Autodesk Inventor part; units mm, degrees
(part 6 of 10)
  spline S17 degree 5 poles (-10.8792, 7.6525) (-10.8768, 7.6467) (-10.8736, 7.6389) (-10.8696, 7.6293) (-10.8648, 7.6178) (-10.8591, 7.6044) (-10.855, 7.5949) (-10.8509, 7.5854) (-10.8468, 7.576) (-10.8427, 7.5666) (-10.8386, 7.5572) (-10.8344, 7.5479) (-10.8303, 7.5386) (-10.8261, 7.5293) (-10.8219, 7.5201) (-10.8177, 7.5109) (-10.8135, 7.5017) (-10.8093, 7.4926) (-10.8051, 7.4835) (-10.8008, 7.4745) (-10.7966, 7.4654) (-10.7923, 7.4565) (-10.788, 7.4475) (-10.7838, 7.4386) (-10.7795, 7.4297) (-10.7751, 7.4209) (-10.7708, 7.4121) (-10.7665, 7.4033) (-10.7621, 7.3946) (-10.7578, 7.3859) (-10.7526, 7.3755) (-10.7473, 7.3651) (-10.742, 7.3548) (-10.7359, 7.3429) (-10.7297, 7.331) (-10.7244, 7.3209) (-10.7191, 7.3109) (-10.7137, 7.3009) (-10.7084, 7.2909) (-10.703, 7.281) (-10.6977, 7.2712) (-10.6914, 7.2597) (-10.6851, 7.2484) (-10.6797, 7.2387) (-10.6734, 7.2275) (-10.667, 7.2164) (-10.6616, 7.2069) (-10.6552, 7.1959) (-10.6489, 7.185) (-10.6434, 7.1757) (-10.6361, 7.1633) (-10.6288, 7.1511) (-10.6224, 7.1405) (-10.6159, 7.13) (-10.6077, 7.1165) (-10.6012, 7.1061) (-10.5948, 7.0959) (-10.5883, 7.0856) (-10.58, 7.0726) (-10.5736, 7.0626) (-10.5671, 7.0526) (-10.5597, 7.0413) (-10.5523, 7.0301) (-10.5467, 7.0218) (-10.5402, 7.0121) (-10.5338, 7.0026) (-10.5282, 6.9944) (-10.5217, 6.985) (-10.5152, 6.9757) (-10.5097, 6.9677) (-10.5032, 6.9585) (-10.4967, 6.9494) (-10.4911, 6.9416) (-10.4846, 6.9326) (-10.4782, 6.9237) (-10.4726, 6.9162) (-10.4662, 6.9074) (-10.4597, 6.8987) (-10.4542, 6.8914) (-10.4477, 6.8828) (-10.4413, 6.8744) (-10.4357, 6.8672) (-10.4293, 6.8589) (-10.4229, 6.8507) (-10.4174, 6.8437) (-10.411, 6.8356) (-10.4046, 6.8277) (-10.3991, 6.8209) (-10.3928, 6.813) (-10.3864, 6.8053) (-10.381, 6.7987) (-10.3747, 6.7911) (-10.3684, 6.7835) (-10.363, 6.7772) (-10.3567, 6.7698) (-10.3504, 6.7625) (-10.3451, 6.7563) (-10.3389, 6.7491) (-10.3326, 6.7421) (-10.3273, 6.7361) (-10.3212, 6.7292) (-10.315, 6.7223) (-10.3098, 6.7166) (-10.3037, 6.7099) (-10.2976, 6.7033) (-10.2924, 6.6977) (-10.2864, 6.6912) (-10.2804, 6.6849) (-10.2753, 6.6795) (-10.2693, 6.6733) (-10.2634, 6.6672) (-10.2583, 6.662) (-10.2525, 6.656) (-10.2467, 6.6501) (-10.2417, 6.6451) (-10.2359, 6.6394) (-10.2302, 6.6338) (-10.2253, 6.629) (-10.2196, 6.6235) (-10.214, 6.6181) (-10.2092, 6.6135) (-10.2036, 6.6082) (-10.1981, 6.6031) (-10.1934, 6.5987) (-10.188, 6.5937) (-10.1826, 6.5887) (-10.178, 6.5846) (-10.1727, 6.5798) (-10.1674, 6.5751) (-10.163, 6.5711) (-10.1578, 6.5666) (-10.1527, 6.5621) (-10.1483, 6.5583) (-10.1433, 6.554) (-10.1383, 6.5498) (-10.1341, 6.5463) (-10.1292, 6.5422) (-10.1243, 6.5382) (-10.1203, 6.5349) (-10.1155, 6.531) (-10.1109, 6.5273) (-10.1069, 6.5241) (-10.1024, 6.5205) (-10.0979, 6.517) (-10.0941, 6.5141) (-10.0898, 6.5107) (-10.0855, 6.5075) (-10.0818, 6.5047) (-10.0777, 6.5016) (-10.0736, 6.4986) (-10.0701, 6.496) (-10.0662, 6.4931) (-10.0623, 6.4903) (-10.059, 6.488) (-10.0558, 6.4857) (-10.0516, 6.4828) (-10.048, 6.4803) (-10.044, 6.4775) (-10.0401, 6.4749) (-10.0363, 6.4724) (-10.0336, 6.4706) (-10.0309, 6.4688) (-10.0287, 6.4674) (-10.0266, 6.466) (-10.0245, 6.4646) (-10.0224, 6.4633) (-10.0204, 6.4621) (-10.0185, 6.4608) (-10.0166, 6.4597) (-10.0147, 6.4585) (-10.0129, 6.4574) (-10.0112, 6.4564) (-10.0095, 6.4553) (-10.0078, 6.4544) (-10.0063, 6.4534) (-10.0047, 6.4525) (-10.0033, 6.4517) (-10.0018, 6.4508) (-10.0005, 6.4501) (-9.9992, 6.4493) (-9.9979, 6.4486) (-9.9967, 6.448) (-9.9956, 6.4473) (-9.9946, 6.4468) (-9.9936, 6.4462) (-9.9926, 6.4457) (-9.9918, 6.4452) (-9.9909, 6.4448) (-9.9902, 6.4444) (-9.9895, 6.4441) (-9.9889, 6.4438) (-9.9883, 6.4434) (-9.9878, 6.4432) (-9.9875, 6.443) (-9.9873, 6.4429) (-9.9872, 6.4429) knots -1 -1 -1 -1 -1 -1 -0.9875 -0.983333 -0.979167 -0.975 -0.970833 -0.966667 -0.9625 -0.958333 -0.954167 -0.95 -0.945833 -0.941667 -0.9375 -0.933333 -0.929167 -0.925 -0.920833 -0.916667 -0.9125 -0.908333 -0.904167 -0.9 -0.895833 -0.891667 -0.8875 -0.883333 -0.879167 -0.875 -0.870833 -0.8625 -0.858333 -0.854167 -0.845833 -0.841667 -0.8375 -0.833333 -0.829167 -0.820833 -0.816667 -0.8125 -0.804167 -0.8 -0.795833 -0.7875 -0.783333 -0.779167 -0.770833 -0.766667 -0.7625 -0.75 -0.745833 -0.741667 -0.7375 -0.725 -0.720833 -0.716667 -0.7125 -0.7 -0.695833 -0.691667 -0.683333 -0.679167 -0.675 -0.666667 -0.6625 -0.658333 -0.65 -0.645833 -0.641667 -0.633333 -0.629167 -0.625 -0.616667 -0.6125 -0.608333 -0.6 -0.595833 -0.591667 -0.583333 -0.579167 -0.575 -0.566667 -0.5625 -0.558333 -0.55 -0.545833 -0.541667 -0.533333 -0.529167 -0.525 -0.516667 -0.5125 -0.508333 -0.5 -0.495833 -0.491667 -0.483333 -0.479167 -0.475 -0.466667 -0.4625 -0.458333 -0.45 -0.445833 -0.441667 -0.433333 -0.429167 -0.425 -0.416667 -0.4125 -0.408333 -0.4 -0.395833 -0.391667 -0.383333 -0.379167 -0.375 -0.366667 -0.3625 -0.358333 -0.35 -0.345833 -0.341667 -0.333333 -0.329167 -0.325 -0.316667 -0.3125 -0.308333 -0.3 -0.295833 -0.291667 -0.283333 -0.279167 -0.275 -0.266667 -0.2625 -0.258333 -0.25 -0.245833 -0.241667 -0.233333 -0.229167 -0.225 -0.216667 -0.2125 -0.208333 -0.2 -0.195833 -0.191667 -0.183333 -0.179167 -0.175 -0.170833 -0.158333 -0.154167 -0.145833 -0.141667 -0.1375 -0.133333 -0.129167 -0.125 -0.120833 -0.116667 -0.1125 -0.108333 -0.104167 -0.1 -0.095833 -0.091667 -0.0875 -0.083333 -0.079167 -0.075 -0.070833 -0.066667 -0.0625 -0.058333 -0.054167 -0.05 -0.045833 -0.041667 -0.0375 -0.033333 -0.029167 -0.025 -0.020833 -0.016667 -0.0125 -0.008333 0 0 0 0 0 0
  line L36 (-8.4168, 7.2079) -> (-9.0752, 7.804)
  arc A18 (-7.5895, 7.9321) -> (-8.4168, 7.2079) centre (-4.8955, 4.02) ccw
  line L37 (-9.0752, 7.804) -> (-9.0757, 7.8044)
  spline S18 degree 5 poles (-9.0757, 7.8044) (-9.0757, 7.8045) (-9.0758, 7.8046) (-9.076, 7.8047) (-9.0763, 7.8049) (-9.0767, 7.8053) (-9.0771, 7.8057) (-9.0777, 7.8061) (-9.0782, 7.8066) (-9.0789, 7.8071) (-9.0796, 7.8077) (-9.0804, 7.8084) (-9.0812, 7.809) (-9.0821, 7.8097) (-9.083, 7.8105) (-9.084, 7.8113) (-9.0851, 7.8122) (-9.0862, 7.813) (-9.0874, 7.814) (-9.0886, 7.8149) (-9.0899, 7.8159) (-9.0913, 7.817) (-9.0927, 7.818) (-9.0942, 7.8191) (-9.0957, 7.8203) (-9.0973, 7.8215) (-9.0989, 7.8227) (-9.1006, 7.8239) (-9.1024, 7.8252) (-9.1042, 7.8265) (-9.1061, 7.8278) (-9.108, 7.8292) (-9.1104, 7.8309) (-9.1129, 7.8326) (-9.1154, 7.8343) (-9.1185, 7.8365) (-9.1217, 7.8386) (-9.1245, 7.8405) (-9.1279, 7.8427) (-9.1314, 7.845) (-9.1345, 7.8471) (-9.1376, 7.8491) (-9.1414, 7.8515) (-9.1464, 7.8547) (-9.1516, 7.8579) (-9.157, 7.8612) (-9.1625, 7.8646) (-9.1683, 7.868) (-9.1728, 7.8707) (-9.1775, 7.8734) (-9.1822, 7.8761) (-9.1878, 7.8793) (-9.1928, 7.8821) (-9.1972, 7.8846) (-9.2023, 7.8874) (-9.2076, 7.8903) (-9.2122, 7.8928) (-9.2176, 7.8957) (-9.2232, 7.8987) (-9.228, 7.9012) (-9.2338, 7.9042) (-9.2396, 7.9072) (-9.2447, 7.9098) (-9.2507, 7.9128) (-9.2568, 7.9159) (-9.2621, 7.9185) (-9.2684, 7.9216) (-9.2748, 7.9246) (-9.2803, 7.9273) (-9.2869, 7.9304) (-9.2935, 7.9335) (-9.2993, 7.9362) (-9.3061, 7.9393) (-9.313, 7.9424) (-9.319, 7.9451) (-9.3261, 7.9483) (-9.3333, 7.9514) (-9.3395, 7.9541) (-9.3468, 7.9572) (-9.3543, 7.9604) (-9.3607, 7.9631) (-9.3683, 7.9662) (-9.376, 7.9694) (-9.3827, 7.9721) (-9.3905, 7.9752) (-9.3985, 7.9784) (-9.4054, 7.981) (-9.4135, 7.9842) (-9.4217, 7.9873) (-9.4287, 7.99) (-9.4371, 7.9931) (-9.4455, 7.9962) (-9.4528, 7.9988) (-9.4614, 8.0019) (-9.4701, 8.005) (-9.4776, 8.0076) (-9.4865, 8.0107) (-9.4954, 8.0137) (-9.5031, 8.0163) (-9.5122, 8.0193) (-9.5213, 8.0223) (-9.5292, 8.0249) (-9.5385, 8.0279) (-9.5479, 8.0308) (-9.556, 8.0334) (-9.5656, 8.0363) (-9.5752, 8.0392) (-9.5835, 8.0417) (-9.5933, 8.0446) (-9.6031, 8.0474) (-9.6116, 8.0498) (-9.6216, 8.0527) (-9.6317, 8.0555) (-9.6404, 8.0578) (-9.6506, 8.0606) (-9.6609, 8.0633) (-9.6697, 8.0656) (-9.6802, 8.0683) (-9.6907, 8.071) (-9.6997, 8.0733) (-9.7104, 8.0759) (-9.7211, 8.0785) (-9.7303, 8.0807) (-9.7412, 8.0832) (-9.7521, 8.0857) (-9.7616, 8.0878) (-9.7726, 8.0903) (-9.7838, 8.0927) (-9.7934, 8.0948) (-9.8046, 8.0972) (-9.816, 8.0995) (-9.8257, 8.1015) (-9.8372, 8.1038) (-9.8488, 8.106) (-9.8587, 8.1079) (-9.8704, 8.1101) (-9.8821, 8.1123) (-9.8922, 8.1141) (-9.9041, 8.1162) (-9.916, 8.1182) (-9.9263, 8.12) (-9.9384, 8.122) (-9.9505, 8.1239) (-9.9609, 8.1256) (-9.9732, 8.1275) (-9.9855, 8.1293) (-9.9961, 8.1309) (-10.0103, 8.1329) (-10.0246, 8.1349) (-10.0372, 8.1366) (-10.0499, 8.1382) (-10.0626, 8.1398) (-10.0772, 8.1417) (-10.0918, 8.1434) (-10.1066, 8.1451) (-10.1215, 8.1467) (-10.1383, 8.1485) (-10.1495, 8.1496) (-10.1608, 8.1507) (-10.1759, 8.1522) (-10.1912, 8.1535) (-10.2045, 8.1547) (-10.218, 8.1558) (-10.2315, 8.1569) (-10.2411, 8.1576) (-10.2508, 8.1583) (-10.2606, 8.159) (-10.2703, 8.1596) (-10.2801, 8.1603) (-10.2899, 8.1609) (-10.2998, 8.1615) (-10.3097, 8.1621) (-10.3196, 8.1626) (-10.3295, 8.1631) (-10.3395, 8.1636) (-10.3494, 8.1641) (-10.3595, 8.1645) (-10.3695, 8.165) (-10.3796, 8.1654) (-10.3897, 8.1657) (-10.3998, 8.1661) (-10.41, 8.1664) (-10.4201, 8.1667) (-10.4304, 8.167) (-10.4406, 8.1672) (-10.4509, 8.1674) (-10.4611, 8.1676) (-10.4715, 8.1678) (-10.4818, 8.1679) (-10.4963, 8.1681) (-10.5088, 8.1682) (-10.5193, 8.1682) (-10.5276, 8.1683) (-10.5339, 8.1683) knots 0 0 0 0 0 0 0.004167 0.008333 0.0125 0.016667 0.020833 0.025 0.029167 0.033333 0.0375 0.041667 0.045833 0.05 0.054167 0.058333 0.0625 0.066667 0.070833 0.075 0.079167 0.083333 0.0875 0.091667 0.095833 0.1 0.104167 0.108333 0.1125 0.116667 0.120833 0.125 0.129167 0.1375 0.141667 0.145833 0.154167 0.158333 0.1625 0.170833 0.175 0.179167 0.183333 0.191667 0.208333 0.2125 0.216667 0.220833 0.229167 0.2375 0.241667 0.245833 0.254167 0.258333 0.2625 0.270833 0.275 0.279167 0.2875 0.291667 0.295833 0.304167 0.308333 0.3125 0.320833 0.325 0.329167 0.3375 0.341667 0.345833 0.354167 0.358333 0.3625 0.370833 0.375 0.379167 0.3875 0.391667 0.395833 0.404167 0.408333 0.4125 0.420833 0.425 0.429167 0.4375 0.441667 0.445833 0.454167 0.458333 0.4625 0.470833 0.475 0.479167 0.4875 0.491667 0.495833 0.504167 0.508333 0.5125 0.520833 0.525 0.529167 0.5375 0.541667 0.545833 0.554167 0.558333 0.5625 0.570833 0.575 0.579167 0.5875 0.591667 0.595833 0.604167 0.608333 0.6125 0.620833 0.625 0.629167 0.6375 0.641667 0.645833 0.654167 0.658333 0.6625 0.670833 0.675 0.679167 0.6875 0.691667 0.695833 0.704167 0.708333 0.7125 0.720833 0.725 0.729167 0.7375 0.741667 0.745833 0.754167 0.758333 0.7625 0.770833 0.775 0.779167 0.791667 0.795833 0.8 0.804167 0.808333 0.825 0.829167 0.833333 0.8375 0.845833 0.85 0.854167 0.866667 0.870833 0.875 0.879167 0.883333 0.8875 0.891667 0.895833 0.9 0.904167 0.908333 0.9125 0.916667 0.920833 0.925 0.929167 0.933333 0.9375 0.941667 0.945833 0.95 0.954167 0.958333 0.9625 0.966667 0.970833 0.975 0.979167 0.983333 0.9875 1 1 1 1 1 1
  arc A19 (-10.5339, 8.1683) -> (-10.8792, 7.6525) centre (-4.8955, 4.02) ccw
  arc A20 (-11.3072, 1.2111) -> (-11.0332, 0.6542) centre (-4.8955, 4.02) ccw
  line L38 (-9.417, 2.5644) -> (-10.2624, 2.2923)
  line L39 (-10.2624, 2.2923) -> (-10.263, 2.2921)
  spline S19 degree 5 poles (-10.263, 2.2921) (-10.2631, 2.292) (-10.2632, 2.292) (-10.2634, 2.2919) (-10.2638, 2.2918) (-10.2643, 2.2916) (-10.2648, 2.2914) (-10.2655, 2.2912) (-10.2662, 2.2909) (-10.267, 2.2906) (-10.2678, 2.2903) (-10.2688, 2.29) (-10.2698, 2.2896) (-10.2708, 2.2892) (-10.2719, 2.2888) (-10.2731, 2.2883) (-10.2744, 2.2878) (-10.2757, 2.2873) (-10.2771, 2.2867) (-10.2786, 2.2861) (-10.2801, 2.2855) (-10.2817, 2.2848) (-10.2833, 2.2841) (-10.285, 2.2834) (-10.2867, 2.2827) (-10.2886, 2.2819) (-10.2904, 2.281) (-10.2924, 2.2802) (-10.2943, 2.2793) (-10.2964, 2.2784) (-10.2985, 2.2774) (-10.3006, 2.2764) (-10.3033, 2.2752) (-10.306, 2.2739) (-10.3088, 2.2726) (-10.3122, 2.271) (-10.3156, 2.2693) (-10.3187, 2.2678) (-10.3223, 2.266) (-10.326, 2.2641) (-10.3293, 2.2625) (-10.3332, 2.2605) (-10.3372, 2.2584) (-10.3407, 2.2565) (-10.3449, 2.2543) (-10.3491, 2.252) (-10.3528, 2.25) (-10.3572, 2.2476) (-10.3617, 2.2451) (-10.3656, 2.2429) (-10.3703, 2.2403) (-10.375, 2.2376) (-10.3791, 2.2352) (-10.3839, 2.2324) (-10.3889, 2.2295) (-10.3932, 2.2269) (-10.3982, 2.2239) (-10.4034, 2.2208) (-10.4078, 2.218) (-10.4131, 2.2148) (-10.4184, 2.2114) (-10.423, 2.2085) (-10.4285, 2.2051) (-10.434, 2.2015) (-10.4388, 2.1984) (-10.4444, 2.1947) (-10.4501, 2.1909) (-10.455, 2.1877) (-10.4608, 2.1837) (-10.4667, 2.1798) (-10.4717, 2.1763) (-10.4777, 2.1722) (-10.4837, 2.168) (-10.4889, 2.1643) (-10.495, 2.1599) (-10.5012, 2.1555) (-10.5065, 2.1517) (-10.5128, 2.1471) (-10.5191, 2.1425) (-10.5245, 2.1384) (-10.5309, 2.1336) (-10.5374, 2.1288) (-10.5429, 2.1245) (-10.5495, 2.1195) (-10.556, 2.1144) (-10.5617, 2.11) (-10.5684, 2.1048) (-10.575, 2.0995) (-10.5808, 2.0949) (-10.5876, 2.0894) (-10.5944, 2.0839) (-10.6002, 2.0791) (-10.6071, 2.0734) (-10.614, 2.0676) (-10.62, 2.0626) (-10.6269, 2.0567) (-10.6339, 2.0508) (-10.64, 2.0456) (-10.647, 2.0394) (-10.6541, 2.0332) (-10.6602, 2.0279) (-10.6674, 2.0215) (-10.6746, 2.0151) (-10.6807, 2.0095) (-10.688, 2.0029) (-10.6952, 1.9963) (-10.7015, 1.9905) (-10.7088, 1.9837) (-10.7161, 1.9769) (-10.7224, 1.9709) (-10.7298, 1.9639) (-10.7372, 1.9568) (-10.7435, 1.9506) (-10.751, 1.9434) (-10.7584, 1.9361) (-10.7648, 1.9297) (-10.7723, 1.9223) (-10.7798, 1.9147) (-10.7863, 1.9082) (-10.7938, 1.9005) (-10.8014, 1.8927) (-10.8079, 1.886) (-10.8154, 1.8781) (-10.823, 1.8701) (-10.8296, 1.8632) (-10.8372, 1.8551) (-10.8448, 1.8469) (-10.8514, 1.8398) (-10.8591, 1.8314) (-10.8667, 1.823) (-10.8733, 1.8157) (-10.881, 1.8071) (-10.8887, 1.7985) (-10.8953, 1.791) (-10.903, 1.7822) (-10.9107, 1.7734) (-10.9174, 1.7657) (-10.9251, 1.7567) (-10.9328, 1.7476) (-10.9395, 1.7397) (-10.9472, 1.7305) (-10.955, 1.7212) (-10.9616, 1.7132) (-10.9694, 1.7037) (-10.9771, 1.6942) (-10.9838, 1.686) (-10.9915, 1.6763) (-10.9993, 1.6666) (-11.0059, 1.6582) (-11.0126, 1.6497) (-11.0226, 1.6369) (-11.0314, 1.6254) (-11.0403, 1.6139) (-11.0492, 1.6022) (-11.0602, 1.5874) (-11.068, 1.577) (-11.0757, 1.5666) (-11.0834, 1.556) (-11.0945, 1.5408) (-11.1033, 1.5286) (-11.1121, 1.5162) (-11.1209, 1.5037) (-11.1297, 1.4911) (-11.1352, 1.4832) (-11.1406, 1.4753) (-11.1461, 1.4673) (-11.1516, 1.4593) (-11.1571, 1.4513) (-11.1625, 1.4432) (-11.168, 1.4351) (-11.1734, 1.4269) (-11.1789, 1.4187) (-11.1843, 1.4105) (-11.1897, 1.4022) (-11.1951, 1.3939) (-11.2006, 1.3856) (-11.206, 1.3772) (-11.2114, 1.3688) (-11.2168, 1.3603) (-11.2222, 1.3518) (-11.2275, 1.3433) (-11.2329, 1.3348) (-11.2383, 1.3262) (-11.2436, 1.3175) (-11.249, 1.3089) (-11.2543, 1.3002) (-11.2597, 1.2914) (-11.265, 1.2826) (-11.2703, 1.2738) (-11.2756, 1.265) (-11.2809, 1.2561) (-11.2883, 1.2436) (-11.2946, 1.2328) (-11.2999, 1.2238) (-11.3041, 1.2166) (-11.3072, 1.2111) knots 0 0 0 0 0 0 0.004167 0.008333 0.0125 0.016667 0.020833 0.025 0.029167 0.033333 0.0375 0.041667 0.045833 0.05 0.054167 0.058333 0.0625 0.066667 0.070833 0.075 0.079167 0.083333 0.0875 0.091667 0.095833 0.1 0.104167 0.108333 0.1125 0.116667 0.120833 0.125 0.129167 0.1375 0.141667 0.145833 0.154167 0.158333 0.1625 0.170833 0.175 0.179167 0.1875 0.191667 0.195833 0.204167 0.208333 0.2125 0.220833 0.225 0.229167 0.2375 0.241667 0.245833 0.254167 0.258333 0.2625 0.270833 0.275 0.279167 0.2875 0.291667 0.295833 0.304167 0.308333 0.3125 0.320833 0.325 0.329167 0.3375 0.341667 0.345833 0.354167 0.358333 0.3625 0.370833 0.375 0.379167 0.3875 0.391667 0.395833 0.404167 0.408333 0.4125 0.420833 0.425 0.429167 0.4375 0.441667 0.445833 0.454167 0.458333 0.4625 0.470833 0.475 0.479167 0.4875 0.491667 0.495833 0.504167 0.508333 0.5125 0.520833 0.525 0.529167 0.5375 0.541667 0.545833 0.554167 0.558333 0.5625 0.570833 0.575 0.579167 0.5875 0.591667 0.595833 0.604167 0.608333 0.6125 0.620833 0.625 0.629167 0.6375 0.641667 0.645833 0.654167 0.658333 0.6625 0.670833 0.675 0.679167 0.6875 0.691667 0.695833 0.704167 0.708333 0.7125 0.720833 0.725 0.729167 0.7375 0.741667 0.745833 0.754167 0.758333 0.7625 0.770833 0.775 0.779167 0.783333 0.8 0.804167 0.808333 0.8125 0.825 0.829167 0.833333 0.8375 0.854167 0.858333 0.8625 0.866667 0.870833 0.875 0.879167 0.883333 0.8875 0.891667 0.895833 0.9 0.904167 0.908333 0.9125 0.916667 0.920833 0.925 0.929167 0.933333 0.9375 0.941667 0.945833 0.95 0.954167 0.958333 0.9625 0.966667 0.970833 0.975 0.979167 0.983333 0.9875 1 1 1 1 1 1
  line L40 (-5.8957, -0.6235) -> (-6.0827, -1.4918)
  line L41 (-6.0827, -1.4918) -> (-6.0828, -1.4924)
  spline S20 degree 5 poles (-6.0828, -1.4924) (-6.0828, -1.4925) (-6.0829, -1.4926) (-6.0829, -1.4928) (-6.083, -1.4932) (-6.0831, -1.4937) (-6.0832, -1.4943) (-6.0833, -1.4949) (-6.0834, -1.4957) (-6.0836, -1.4965) (-6.0837, -1.4974) (-6.0839, -1.4984) (-6.0841, -1.4994) (-6.0842, -1.5006) (-6.0844, -1.5018) (-6.0846, -1.503) (-6.0848, -1.5044) (-6.085, -1.5058) (-6.0852, -1.5073) (-6.0854, -1.5088) (-6.0857, -1.5105) (-6.0859, -1.5121) (-6.0861, -1.5139) (-6.0863, -1.5157) (-6.0866, -1.5176) (-6.0868, -1.5196) (-6.087, -1.5216) (-6.0872, -1.5237) (-6.0875, -1.5259) (-6.0877, -1.5281) (-6.0879, -1.5304) (-6.0881, -1.5328) (-6.0884, -1.5357) (-6.0886, -1.5387) (-6.0889, -1.5418) (-6.0892, -1.5455) (-6.0894, -1.5493) (-6.0897, -1.5527) (-6.0899, -1.5568) (-6.0902, -1.5609) (-6.0904, -1.5646) (-6.0906, -1.569) (-6.0908, -1.5735) (-6.0909, -1.5774) (-6.0911, -1.5822) (-6.0912, -1.587) (-6.0913, -1.5912) (-6.0914, -1.5962) (-6.0915, -1.6014) (-6.0916, -1.6058) (-6.0916, -1.6112) (-6.0917, -1.6166) (-6.0916, -1.6213) (-6.0916, -1.6269) (-6.0916, -1.6327) (-6.0915, -1.6377) (-6.0914, -1.6436) (-6.0913, -1.6496) (-6.0911, -1.6548) (-6.0909, -1.661) (-6.0907, -1.6673) (-6.0905, -1.6727) (-6.0902, -1.6792) (-6.0899, -1.6857) (-6.0896, -1.6914) (-6.0892, -1.6981) (-6.0888, -1.7049) (-6.0884, -1.7109) (-6.0879, -1.7178) (-6.0874, -1.7249) (-6.0869, -1.731) (-6.0863, -1.7382) (-6.0857, -1.7456) (-6.0851, -1.7519) (-6.0844, -1.7594) (-6.0837, -1.7669) (-6.083, -1.7735) (-6.0822, -1.7812) (-6.0813, -1.789) (-6.0805, -1.7957) (-6.0796, -1.8036) (-6.0786, -1.8116) (-6.0777, -1.8186) (-6.0766, -1.8267) (-6.0755, -1.835) (-6.0745, -1.8421) (-6.0733, -1.8504) (-6.0721, -1.8589) (-6.0709, -1.8662) (-6.0696, -1.8748) (-6.0682, -1.8834) (-6.067, -1.8909) (-6.0655, -1.8997) (-6.064, -1.9086) (-6.0626, -1.9162) (-6.061, -1.9252) (-6.0593, -1.9343) (-6.0578, -1.9421) (-6.0561, -1.9512) (-6.0542, -1.9605) (-6.0526, -1.9685) (-6.0507, -1.9778) (-6.0487, -1.9873) (-6.047, -1.9954) (-6.0449, -2.005) (-6.0428, -2.0146) (-6.0409, -2.0229) (-6.0387, -2.0326) (-6.0364, -2.0424) (-6.0344, -2.0508) (-6.032, -2.0607) (-6.0295, -2.0706) (-6.0274, -2.0792) (-6.0248, -2.0893) (-6.0222, -2.0994) (-6.0199, -2.1081) (-6.0172, -2.1183) (-6.0145, -2.1286) (-6.012, -2.1375) (-6.0091, -2.1478) (-6.0062, -2.1583) (-6.0036, -2.1672) (-6.0006, -2.1778) (-5.9974, -2.1884) (-5.9947, -2.1975) (-5.9915, -2.2081) (-5.9882, -2.2188) (-5.9853, -2.2281) (-5.9819, -2.2389) (-5.9785, -2.2497) (-5.9755, -2.2591) (-5.9719, -2.27) (-5.9682, -2.281) (-5.9651, -2.2905) (-5.9613, -2.3016) (-5.9575, -2.3127) (-5.9542, -2.3223) (-5.9502, -2.3335) (-5.9462, -2.3447) (-5.9427, -2.3544) (-5.9386, -2.3657) (-5.9344, -2.3771) (-5.9308, -2.3868) (-5.9265, -2.3983) (-5.9221, -2.4098) (-5.9183, -2.4196) (-5.9138, -2.4312) (-5.9093, -2.4428) (-5.9053, -2.4527) (-5.9013, -2.4627) (-5.8952, -2.4778) (-5.8897, -2.4912) (-5.8841, -2.5046) (-5.8785, -2.5181) (-5.8712, -2.5351) (-5.8661, -2.547) (-5.8609, -2.5589) (-5.8556, -2.5709) (-5.8487, -2.5863) (-5.8433, -2.5984) (-5.8378, -2.6105) (-5.8315, -2.6243) (-5.825, -2.6382) (-5.8201, -2.6486) (-5.8152, -2.6591) (-5.8102, -2.6695) (-5.8059, -2.6783) (-5.8017, -2.687) (-5.7974, -2.6958) (-5.7931, -2.7046) (-5.7888, -2.7134) (-5.7844, -2.7222) (-5.78, -2.731) (-5.7756, -2.7399) (-5.7711, -2.7487) (-5.7666, -2.7576) (-5.762, -2.7664) (-5.7574, -2.7753) (-5.7528, -2.7842) (-5.7482, -2.7931) (-5.7435, -2.8021) (-5.7387, -2.811) (-5.734, -2.8199) (-5.7292, -2.8289) (-5.7243, -2.8379) (-5.7195, -2.8468) (-5.7146, -2.8558) (-5.7096, -2.8648) (-5.7046, -2.8738) (-5.6996, -2.8828) (-5.6946, -2.8919) (-5.6875, -2.9045) (-5.6813, -2.9154) (-5.6761, -2.9245) (-5.672, -2.9317) (-5.6688, -2.9372) knots 0 0 0 0 0 0 0.004167 0.008333 0.0125 0.016667 0.020833 0.025 0.029167 0.033333 0.0375 0.041667 0.045833 0.05 0.054167 0.058333 0.0625 0.066667 0.070833 0.075 0.079167 0.083333 0.0875 0.091667 0.095833 0.1 0.104167 0.108333 0.1125 0.116667 0.120833 0.125 0.129167 0.1375 0.141667 0.145833 0.154167 0.158333 0.1625 0.170833 0.175 0.179167 0.1875 0.191667 0.195833 0.204167 0.208333 0.2125 0.220833 0.225 0.229167 0.2375 0.241667 0.245833 0.254167 0.258333 0.2625 0.270833 0.275 0.279167 0.2875 0.291667 0.295833 0.304167 0.308333 0.3125 0.320833 0.325 0.329167 0.3375 0.341667 0.345833 0.354167 0.358333 0.3625 0.370833 0.375 0.379167 0.3875 0.391667 0.395833 0.404167 0.408333 0.4125 0.420833 0.425 0.429167 0.4375 0.441667 0.445833 0.454167 0.458333 0.4625 0.470833 0.475 0.479167 0.4875 0.491667 0.495833 0.504167 0.508333 0.5125 0.520833 0.525 0.529167 0.5375 0.541667 0.545833 0.554167 0.558333 0.5625 0.570833 0.575 0.579167 0.5875 0.591667 0.595833 0.604167 0.608333 0.6125 0.620833 0.625 0.629167 0.6375 0.641667 0.645833 0.654167 0.658333 0.6625 0.670833 0.675 0.679167 0.6875 0.691667 0.695833 0.704167 0.708333 0.7125 0.720833 0.725 0.729167 0.7375 0.741667 0.745833 0.754167 0.758333 0.7625 0.770833 0.775 0.779167 0.783333 0.8 0.804167 0.808333 0.8125 0.825 0.829167 0.833333 0.8375 0.85 0.854167 0.858333 0.866667 0.870833 0.875 0.879167 0.883333 0.8875 0.891667 0.895833 0.9 0.904167 0.908333 0.9125 0.916667 0.920833 0.925 0.929167 0.933333 0.9375 0.941667 0.945833 0.95 0.954167 0.958333 0.9625 0.966667 0.970833 0.975 0.979167 0.983333 0.9875 1 1 1 1 1 1
  arc A21 (-5.6688, -2.9372) -> (-5.0495, -2.9783) centre (-4.8955, 4.02) ccw
  line L42 (-4.448, -1.6004) -> (-4.5185, -0.715)
  line L43 (-4.4479, -1.601) -> (-4.448, -1.6004)
  spline S21 degree 5 poles (-5.0495, -2.9783) (-5.0456, -2.9733) (-5.0405, -2.9667) (-5.0342, -2.9584) (-5.0267, -2.9484) (-5.0179, -2.9368) (-5.0117, -2.9286) (-5.0056, -2.9203) (-4.9994, -2.912) (-4.9934, -2.9037) (-4.9873, -2.8955) (-4.9813, -2.8872) (-4.9753, -2.879) (-4.9694, -2.8707) (-4.9635, -2.8625) (-4.9576, -2.8543) (-4.9518, -2.846) (-4.946, -2.8378) (-4.9402, -2.8296) (-4.9345, -2.8214) (-4.9288, -2.8132) (-4.9232, -2.805) (-4.9175, -2.7969) (-4.912, -2.7887) (-4.9064, -2.7805) (-4.9009, -2.7724) (-4.8955, -2.7642) (-4.89, -2.7561) (-4.8846, -2.748) (-4.8793, -2.7398) (-4.8729, -2.7301) (-4.8666, -2.7204) (-4.8603, -2.7107) (-4.853, -2.6994) (-4.8459, -2.6881) (-4.8397, -2.6785) (-4.8337, -2.6688) (-4.8277, -2.6592) (-4.8218, -2.6496) (-4.8159, -2.64) (-4.81, -2.6304) (-4.8033, -2.6193) (-4.7966, -2.6082) (-4.7909, -2.5986) (-4.7844, -2.5876) (-4.7779, -2.5765) (-4.7724, -2.5671) (-4.7661, -2.556) (-4.7598, -2.5451) (-4.7545, -2.5357) (-4.7483, -2.5248) (-4.7422, -2.5139) (-4.7371, -2.5045) (-4.7303, -2.4921) (-4.7236, -2.4798) (-4.7178, -2.469) (-4.7121, -2.4583) (-4.7048, -2.4445) (-4.6993, -2.4338) (-4.6938, -2.4232) (-4.6883, -2.4126) (-4.6815, -2.399) (-4.6762, -2.3885) (-4.671, -2.378) (-4.6651, -2.3661) (-4.6594, -2.3542) (-4.6551, -2.3453) (-4.6502, -2.335) (-4.6453, -2.3247) (-4.6412, -2.3159) (-4.6365, -2.3057) (-4.6318, -2.2955) (-4.6279, -2.2868) (-4.6234, -2.2767) (-4.6189, -2.2666) (-4.6151, -2.258) (-4.6108, -2.2481) (-4.6065, -2.2381) (-4.6029, -2.2296) (-4.5987, -2.2198) (-4.5946, -2.21) (-4.5912, -2.2016) (-4.5872, -2.1919) (-4.5833, -2.1822) (-4.58, -2.174) (-4.5762, -2.1644) (-4.5725, -2.1549) (-4.5693, -2.1468) (-4.5657, -2.1373) (-4.5622, -2.1279) (-4.5592, -2.1199) (-4.5557, -2.1107) (-4.5524, -2.1014) (-4.5495, -2.0936) (-4.5463, -2.0844) (-4.5431, -2.0754) (-4.5404, -2.0676) (-4.5373, -2.0587) (-4.5343, -2.0498) (-4.5318, -2.0422) (-4.5289, -2.0334) (-4.526, -2.0246) (-4.5237, -2.0172) (-4.5209, -2.0086) (-4.5182, -2) (-4.516, -1.9927) (-4.5134, -1.9843) (-4.5109, -1.9759) (-4.5088, -1.9688) (-4.5064, -1.9605) (-4.5041, -1.9523) (-4.5021, -1.9454) (-4.4999, -1.9373) (-4.4977, -1.9293) (-4.4959, -1.9225) (-4.4938, -1.9147) (-4.4918, -1.9069) (-4.4901, -1.9003) (-4.4881, -1.8926) (-4.4863, -1.885) (-4.4847, -1.8786) (-4.4829, -1.8711) (-4.4812, -1.8638) (-4.4798, -1.8575) (-4.4781, -1.8503) (-4.4765, -1.8432) (-4.4752, -1.8371) (-4.4737, -1.8301) (-4.4723, -1.8232) (-4.4711, -1.8173) (-4.4698, -1.8106) (-4.4685, -1.8039) (-4.4674, -1.7983) (-4.4662, -1.7917) (-4.465, -1.7853) (-4.464, -1.7799) (-4.463, -1.7736) (-4.4619, -1.7674) (-4.4611, -1.7622) (-4.4601, -1.7562) (-4.4592, -1.7503) (-4.4584, -1.7453) (-4.4576, -1.7396) (-4.4568, -1.734) (-4.4561, -1.7292) (-4.4554, -1.7237) (-4.4547, -1.7184) (-4.4542, -1.7139) (-4.4536, -1.7087) (-4.453, -1.7036) (-4.4525, -1.6994) (-4.452, -1.6945) (-4.4515, -1.6897) (-4.4511, -1.6857) (-4.4507, -1.6818) (-4.4503, -1.6767) (-4.4499, -1.6724) (-4.4496, -1.6675) (-4.4492, -1.6628) (-4.4489, -1.6583) (-4.4487, -1.655) (-4.4485, -1.6518) (-4.4484, -1.6492) (-4.4483, -1.6467) (-4.4481, -1.6442) (-4.448, -1.6417) (-4.4479, -1.6394) (-4.4479, -1.6371) (-4.4478, -1.6348) (-4.4477, -1.6327) (-4.4477, -1.6306) (-4.4476, -1.6285) (-4.4476, -1.6265) (-4.4476, -1.6246) (-4.4475, -1.6228) (-4.4475, -1.621) (-4.4475, -1.6193) (-4.4475, -1.6177) (-4.4475, -1.6161) (-4.4475, -1.6146) (-4.4475, -1.6132) (-4.4476, -1.6118) (-4.4476, -1.6105) (-4.4476, -1.6093) (-4.4476, -1.6082) (-4.4477, -1.6071) (-4.4477, -1.6061) (-4.4477, -1.6052) (-4.4478, -1.6044) (-4.4478, -1.6036) (-4.4478, -1.6029) (-4.4479, -1.6022) (-4.4479, -1.6017) (-4.4479, -1.6014) (-4.4479, -1.6011) (-4.4479, -1.601) knots -1 -1 -1 -1 -1 -1 -0.9875 -0.983333 -0.979167 -0.975 -0.970833 -0.966667 -0.9625 -0.958333 -0.954167 -0.95 -0.945833 -0.941667 -0.9375 -0.933333 -0.929167 -0.925 -0.920833 -0.916667 -0.9125 -0.908333 -0.904167 -0.9 -0.895833 -0.891667 -0.8875 -0.883333 -0.879167 -0.875 -0.870833 -0.8625 -0.858333 -0.854167 -0.845833 -0.841667 -0.8375 -0.833333 -0.829167 -0.820833 -0.816667 -0.8125 -0.804167 -0.8 -0.795833 -0.7875 -0.783333 -0.779167 -0.770833 -0.766667 -0.7625 -0.754167 -0.75 -0.745833 -0.733333 -0.729167 -0.725 -0.720833 -0.708333 -0.704167 -0.7 -0.695833 -0.683333 -0.679167 -0.675 -0.666667 -0.6625 -0.658333 -0.65 -0.645833 -0.641667 -0.633333 -0.629167 -0.625 -0.616667 -0.6125 -0.608333 -0.6 -0.595833 -0.591667 -0.583333 -0.579167 -0.575 -0.566667 -0.5625 -0.558333 -0.55 -0.545833 -0.541667 -0.533333 -0.529167 -0.525 -0.516667 -0.5125 -0.508333 -0.5 -0.495833 -0.491667 -0.483333 -0.479167 -0.475 -0.466667 -0.4625 -0.458333 -0.45 -0.445833 -0.441667 -0.433333 -0.429167 -0.425 -0.416667 -0.4125 -0.408333 -0.4 -0.395833 -0.391667 -0.383333 -0.379167 -0.375 -0.366667 -0.3625 -0.358333 -0.35 -0.345833 -0.341667 -0.333333 -0.329167 -0.325 -0.316667 -0.3125 -0.308333 -0.3 -0.295833 -0.291667 -0.283333 -0.279167 -0.275 -0.266667 -0.2625 -0.258333 -0.25 -0.245833 -0.241667 -0.233333 -0.229167 -0.225 -0.216667 -0.2125 -0.208333 -0.2 -0.195833 -0.191667 -0.183333 -0.179167 -0.175 -0.170833 -0.158333 -0.154167 -0.145833 -0.141667 -0.1375 -0.133333 -0.129167 -0.125 -0.120833 -0.116667 -0.1125 -0.108333 -0.104167 -0.1 -0.095833 -0.091667 -0.0875 -0.083333 -0.079167 -0.075 -0.070833 -0.066667 -0.0625 -0.058333 -0.054167 -0.05 -0.045833 -0.041667 -0.0375 -0.033333 -0.029167 -0.025 -0.020833 -0.016667 -0.0125 -0.008333 0 0 0 0 0 0
  arc A22 (-4.5185, -0.715) -> (-3.4399, -0.5015) centre (-4.8955, 4.02) ccw
  line L44 (-3.4399, -0.5015) -> (-3.1678, -1.3469)
  line L45 (-3.1678, -1.3469) -> (-3.1676, -1.3475)
  line L46 (-1.6978, -0.6236) -> (-2.2015, 0.1079)
  line L47 (-1.6974, -0.6242) -> (-1.6978, -0.6236)
  spline S22 degree 5 poles (-3.1676, -1.3475) (-3.1675, -1.3476) (-3.1675, -1.3477) (-3.1674, -1.3479) (-3.1673, -1.3483) (-3.1671, -1.3488) (-3.1669, -1.3493) (-3.1667, -1.35) (-3.1664, -1.3507) (-3.1662, -1.3515) (-3.1658, -1.3523) (-3.1655, -1.3533) (-3.1651, -1.3543) (-3.1647, -1.3553) (-3.1643, -1.3565) (-3.1638, -1.3577) (-3.1633, -1.3589) (-3.1628, -1.3602) (-3.1622, -1.3616) (-3.1616, -1.3631) (-3.161, -1.3646) (-3.1603, -1.3662) (-3.1596, -1.3678) (-3.1589, -1.3695) (-3.1582, -1.3713) (-3.1574, -1.3731) (-3.1566, -1.3749) (-3.1557, -1.3769) (-3.1548, -1.3789) (-3.1539, -1.3809) (-3.153, -1.383) (-3.152, -1.3851) (-3.1507, -1.3878) (-3.1495, -1.3905) (-3.1481, -1.3933) (-3.1465, -1.3967) (-3.1448, -1.4001) (-3.1433, -1.4032) (-3.1415, -1.4068) (-3.1396, -1.4106) (-3.138, -1.4138) (-3.136, -1.4177) (-3.1339, -1.4217) (-3.132, -1.4252) (-3.1298, -1.4294) (-3.1275, -1.4337) (-3.1255, -1.4374) (-3.1231, -1.4418) (-3.1206, -1.4463) (-3.1184, -1.4502) (-3.1158, -1.4548) (-3.1131, -1.4595) (-3.1107, -1.4636) (-3.1079, -1.4685) (-3.105, -1.4734) (-3.1024, -1.4777) (-3.0994, -1.4827) (-3.0963, -1.4879) (-3.0935, -1.4923) (-3.0903, -1.4976) (-3.087, -1.5029) (-3.084, -1.5075) (-3.0806, -1.513) (-3.077, -1.5185) (-3.0739, -1.5233) (-3.0702, -1.5289) (-3.0665, -1.5346) (-3.0632, -1.5395) (-3.0593, -1.5453) (-3.0553, -1.5512) (-3.0518, -1.5563) (-3.0477, -1.5622) (-3.0435, -1.5682) (-3.0398, -1.5734) (-3.0355, -1.5795) (-3.031, -1.5857) (-3.0272, -1.591) (-3.0226, -1.5973) (-3.018, -1.6036) (-3.0139, -1.6091) (-3.0092, -1.6155) (-3.0043, -1.6219) (-3.0001, -1.6275) (-2.995, -1.634) (-2.99, -1.6406) (-2.9855, -1.6462) (-2.9803, -1.6529) (-2.975, -1.6596) (-2.9704, -1.6653) (-2.9649, -1.6721) (-2.9594, -1.6789) (-2.9546, -1.6847) (-2.9489, -1.6916) (-2.9431, -1.6985) (-2.9382, -1.7045) (-2.9323, -1.7114) (-2.9263, -1.7184) (-2.9211, -1.7245) (-2.915, -1.7315) (-2.9088, -1.7386) (-2.9034, -1.7447) (-2.897, -1.7519) (-2.8906, -1.7591) (-2.885, -1.7652) (-2.8785, -1.7725) (-2.8718, -1.7797) (-2.866, -1.786) (-2.8592, -1.7933) (-2.8524, -1.8006) (-2.8464, -1.8069) (-2.8394, -1.8143) (-2.8323, -1.8217) (-2.8262, -1.828) (-2.8189, -1.8355) (-2.8116, -1.8429) (-2.8053, -1.8493) (-2.7978, -1.8568) (-2.7902, -1.8643) (-2.7837, -1.8708) (-2.776, -1.8783) (-2.7683, -1.8859) (-2.7615, -1.8924) (-2.7536, -1.9) (-2.7456, -1.9076) (-2.7387, -1.9141) (-2.7306, -1.9217) (-2.7224, -1.9294) (-2.7153, -1.9359) (-2.7069, -1.9436) (-2.6985, -1.9512) (-2.6912, -1.9578) (-2.6827, -1.9655) (-2.674, -1.9732) (-2.6665, -1.9798) (-2.6577, -1.9875) (-2.6489, -1.9953) (-2.6412, -2.0019) (-2.6322, -2.0096) (-2.6231, -2.0174) (-2.6153, -2.024) (-2.606, -2.0317) (-2.5967, -2.0395) (-2.5887, -2.0461) (-2.5792, -2.0539) (-2.5697, -2.0616) (-2.5615, -2.0683) (-2.5518, -2.0761) (-2.5421, -2.0838) (-2.5337, -2.0905) (-2.5252, -2.0971) (-2.5124, -2.1071) (-2.501, -2.116) (-2.4894, -2.1248) (-2.4777, -2.1337) (-2.463, -2.1447) (-2.4526, -2.1525) (-2.4421, -2.1602) (-2.4315, -2.168) (-2.4163, -2.179) (-2.4041, -2.1878) (-2.3917, -2.1966) (-2.3792, -2.2054) (-2.3667, -2.2142) (-2.3588, -2.2197) (-2.3508, -2.2252) (-2.3429, -2.2306) (-2.3348, -2.2361) (-2.3268, -2.2416) (-2.3187, -2.247) (-2.3106, -2.2525) (-2.3024, -2.2579) (-2.2942, -2.2634) (-2.286, -2.2688) (-2.2777, -2.2742) (-2.2694, -2.2797) (-2.2611, -2.2851) (-2.2527, -2.2905) (-2.2443, -2.2959) (-2.2358, -2.3013) (-2.2274, -2.3067) (-2.2188, -2.3121) (-2.2103, -2.3174) (-2.2017, -2.3228) (-2.193, -2.3281) (-2.1844, -2.3335) (-2.1757, -2.3388) (-2.1669, -2.3442) (-2.1581, -2.3495) (-2.1493, -2.3548) (-2.1405, -2.3601) (-2.1316, -2.3654) (-2.1191, -2.3728) (-2.1083, -2.3791) (-2.0993, -2.3844) (-2.0921, -2.3886) (-2.0866, -2.3917) knots 0 0 0 0 0 0 0.004167 0.008333 0.0125 0.016667 0.020833 0.025 0.029167 0.033333 0.0375 0.041667 0.045833 0.05 0.054167 0.058333 0.0625 0.066667 0.070833 0.075 0.079167 0.083333 0.0875 0.091667 0.095833 0.1 0.104167 0.108333 0.1125 0.116667 0.120833 0.125 0.129167 0.1375 0.141667 0.145833 0.154167 0.158333 0.1625 0.170833 0.175 0.179167 0.1875 0.191667 0.195833 0.204167 0.208333 0.2125 0.220833 0.225 0.229167 0.2375 0.241667 0.245833 0.254167 0.258333 0.2625 0.270833 0.275 0.279167 0.2875 0.291667 0.295833 0.304167 0.308333 0.3125 0.320833 0.325 0.329167 0.3375 0.341667 0.345833 0.354167 0.358333 0.3625 0.370833 0.375 0.379167 0.3875 0.391667 0.395833 0.404167 0.408333 0.4125 0.420833 0.425 0.429167 0.4375 0.441667 0.445833 0.454167 0.458333 0.4625 0.470833 0.475 0.479167 0.4875 0.491667 0.495833 0.504167 0.508333 0.5125 0.520833 0.525 0.529167 0.5375 0.541667 0.545833 0.554167 0.558333 0.5625 0.570833 0.575 0.579167 0.5875 0.591667 0.595833 0.604167 0.608333 0.6125 0.620833 0.625 0.629167 0.6375 0.641667 0.645833 0.654167 0.658333 0.6625 0.670833 0.675 0.679167 0.6875 0.691667 0.695833 0.704167 0.708333 0.7125 0.720833 0.725 0.729167 0.7375 0.741667 0.745833 0.754167 0.758333 0.7625 0.770833 0.775 0.779167 0.783333 0.8 0.804167 0.808333 0.8125 0.825 0.829167 0.833333 0.8375 0.854167 0.858333 0.8625 0.866667 0.870833 0.875 0.879167 0.883333 0.8875 0.891667 0.895833 0.9 0.904167 0.908333 0.9125 0.916667 0.920833 0.925 0.929167 0.933333 0.9375 0.941667 0.945833 0.95 0.954167 0.958333 0.9625 0.966667 0.970833 0.975 0.979167 0.983333 0.9875 1 1 1 1 1 1
  arc A23 (-2.0866, -2.3917) -> (-1.5297, -2.1177) centre (-4.8955, 4.02) ccw
  spline S23 degree 5 poles (-1.5297, -2.1177) (-1.5289, -2.1115) (-1.5278, -2.1032) (-1.5264, -2.0928) (-1.5249, -2.0804) (-1.5231, -2.066) (-1.5219, -2.0557) (-1.5207, -2.0455) (-1.5195, -2.0353) (-1.5184, -2.0251) (-1.5173, -2.0149) (-1.5162, -2.0047) (-1.5151, -1.9946) (-1.5141, -1.9845) (-1.5131, -1.9744) (-1.5122, -1.9643) (-1.5112, -1.9543) (-1.5103, -1.9443) (-1.5094, -1.9343) (-1.5086, -1.9243) (-1.5077, -1.9144) (-1.5069, -1.9045) (-1.5062, -1.8946) (-1.5054, -1.8847) (-1.5047, -1.8749) (-1.504, -1.8651) (-1.5034, -1.8553) (-1.5027, -1.8455) (-1.5021, -1.8358) (-1.5015, -1.8261) (-1.5009, -1.8145) (-1.5003, -1.8029) (-1.4997, -1.7914) (-1.499, -1.7779) (-1.4985, -1.7646) (-1.498, -1.7532) (-1.4976, -1.7418) (-1.4972, -1.7305) (-1.4969, -1.7192) (-1.4965, -1.7079) (-1.4963, -1.6967) (-1.496, -1.6837) (-1.4958, -1.6707) (-1.4956, -1.6596) (-1.4955, -1.6468) (-1.4954, -1.6339) (-1.4954, -1.623) (-1.4954, -1.6103) (-1.4954, -1.5977) (-1.4955, -1.5869) (-1.4957, -1.5725) (-1.4959, -1.5583) (-1.4961, -1.5459) (-1.4964, -1.5336) (-1.4969, -1.5178) (-1.4973, -1.5056) (-1.4977, -1.4934) (-1.4982, -1.4814) (-1.4989, -1.4659) (-1.4994, -1.454) (-1.5001, -1.4421) (-1.5007, -1.4303) (-1.5016, -1.4153) (-1.5024, -1.4036) (-1.5032, -1.392) (-1.5042, -1.3789) (-1.5052, -1.3658) (-1.506, -1.356) (-1.5069, -1.3447) (-1.5079, -1.3335) (-1.5088, -1.3239) (-1.5099, -1.3128) (-1.511, -1.3017) (-1.512, -1.2923) (-1.5132, -1.2814) (-1.5144, -1.2706) (-1.5154, -1.2613) (-1.5167, -1.2506) (-1.518, -1.24) (-1.5192, -1.2309) (-1.5205, -1.2204) (-1.5219, -1.21) (-1.5232, -1.2011) (-1.5246, -1.1908) (-1.5261, -1.1806) (-1.5274, -1.1719) (-1.529, -1.1618) (-1.5305, -1.1518) (-1.5319, -1.1433) (-1.5336, -1.1334) (-1.5352, -1.1236) (-1.5367, -1.1153) (-1.5384, -1.1056) (-1.5401, -1.0961) (-1.5416, -1.0879) (-1.5434, -1.0785) (-1.5452, -1.0692) (-1.5468, -1.0612) (-1.5486, -1.0521) (-1.5505, -1.043) (-1.5521, -1.0352) (-1.554, -1.0263) (-1.556, -1.0174) (-1.5577, -1.0099) (-1.5596, -1.0011) (-1.5616, -0.9925) (-1.5633, -0.9852) (-1.5654, -0.9767) (-1.5674, -0.9683) (-1.5692, -0.9612) (-1.5712, -0.953) (-1.5733, -0.9448) (-1.5751, -0.9379) (-1.5772, -0.93) (-1.5794, -0.9221) (-1.5812, -0.9154) (-1.5833, -0.9076) (-1.5855, -0.9) (-1.5873, -0.8935) (-1.5895, -0.8861) (-1.5917, -0.8787) (-1.5936, -0.8725) (-1.5958, -0.8653) (-1.598, -0.8582) (-1.5998, -0.8521) (-1.602, -0.8452) (-1.6043, -0.8384) (-1.6062, -0.8326) (-1.6084, -0.8259) (-1.6106, -0.8193) (-1.6125, -0.8138) (-1.6147, -0.8074) (-1.6169, -0.8011) (-1.6188, -0.7958) (-1.621, -0.7897) (-1.6232, -0.7837) (-1.625, -0.7786) (-1.6272, -0.7728) (-1.6294, -0.7671) (-1.6313, -0.7623) (-1.6334, -0.7567) (-1.6356, -0.7513) (-1.6374, -0.7467) (-1.6395, -0.7415) (-1.6416, -0.7364) (-1.6434, -0.732) (-1.6455, -0.7271) (-1.6475, -0.7223) (-1.6493, -0.7182) (-1.651, -0.7142) (-1.653, -0.7097) (-1.6547, -0.7059) (-1.6564, -0.7022) (-1.6581, -0.6985) (-1.6602, -0.6938) (-1.6621, -0.6897) (-1.664, -0.6858) (-1.6661, -0.6815) (-1.6681, -0.6773) (-1.6696, -0.6743) (-1.6711, -0.6713) (-1.6725, -0.6685) (-1.6737, -0.6661) (-1.6749, -0.6638) (-1.676, -0.6616) (-1.6771, -0.6595) (-1.6782, -0.6574) (-1.6793, -0.6554) (-1.6804, -0.6534) (-1.6814, -0.6515) (-1.6824, -0.6496) (-1.6834, -0.6478) (-1.6843, -0.6461) (-1.6853, -0.6444) (-1.6862, -0.6428) (-1.687, -0.6413) (-1.6879, -0.6398) (-1.6887, -0.6384) (-1.6895, -0.637) (-1.6903, -0.6357) (-1.691, -0.6345) (-1.6917, -0.6333) (-1.6923, -0.6322) (-1.693, -0.6312) (-1.6936, -0.6302) (-1.6941, -0.6293) (-1.6946, -0.6285) (-1.6951, -0.6277) (-1.6956, -0.627) (-1.696, -0.6263) (-1.6963, -0.6258) (-1.6967, -0.6252) (-1.697, -0.6247) (-1.6972, -0.6245) (-1.6973, -0.6243) (-1.6974, -0.6242) knots -1 -1 -1 -1 -1 -1 -0.9875 -0.983333 -0.979167 -0.975 -0.970833 -0.966667 -0.9625 -0.958333 -0.954167 -0.95 -0.945833 -0.941667 -0.9375 -0.933333 -0.929167 -0.925 -0.920833 -0.916667 -0.9125 -0.908333 -0.904167 -0.9 -0.895833 -0.891667 -0.8875 -0.883333 -0.879167 -0.875 -0.870833 -0.8625 -0.858333 -0.854167 -0.845833 -0.841667 -0.8375 -0.833333 -0.829167 -0.820833 -0.816667 -0.8125 -0.804167 -0.8 -0.795833 -0.7875 -0.783333 -0.779167 -0.770833 -0.766667 -0.7625 -0.75 -0.745833 -0.741667 -0.7375 -0.725 -0.720833 -0.716667 -0.7125 -0.7 -0.695833 -0.691667 -0.6875 -0.675 -0.670833 -0.666667 -0.658333 -0.654167 -0.65 -0.641667 -0.6375 -0.633333 -0.625 -0.620833 -0.616667 -0.608333 -0.604167 -0.6 -0.591667 -0.5875 -0.583333 -0.575 -0.570833 -0.566667 -0.558333 -0.554167 -0.55 -0.541667 -0.5375 -0.533333 -0.525 -0.520833 -0.516667 -0.508333 -0.504167 -0.5 -0.491667 -0.4875 -0.483333 -0.475 -0.470833 -0.466667 -0.458333 -0.454167 -0.45 -0.441667 -0.4375 -0.433333 -0.425 -0.420833 -0.416667 -0.408333 -0.404167 -0.4 -0.391667 -0.3875 -0.383333 -0.375 -0.370833 -0.366667 -0.358333 -0.354167 -0.35 -0.341667 -0.3375 -0.333333 -0.325 -0.320833 -0.316667 -0.308333 -0.304167 -0.3 -0.291667 -0.2875 -0.283333 -0.275 -0.270833 -0.266667 -0.258333 -0.254167 -0.25 -0.241667 -0.2375 -0.233333 -0.225 -0.220833 -0.216667 -0.208333 -0.204167 -0.2 -0.195833 -0.1875 -0.183333 -0.179167 -0.175 -0.1625 -0.158333 -0.154167 -0.145833 -0.141667 -0.1375 -0.133333 -0.129167 -0.125 -0.120833 -0.116667 -0.1125 -0.108333 -0.104167 -0.1 -0.095833 -0.091667 -0.0875 -0.083333 -0.079167 -0.075 -0.070833 -0.066667 -0.0625 -0.058333 -0.054167 -0.05 -0.045833 -0.041667 -0.0375 -0.033333 -0.029167 -0.025 -0.020833 -0.016667 -0.0125 -0.008333 0 0 0 0 0 0
  point P0 (-4.8955, 4.02)
sketch "Sketch1" plane through (0, 0, 0) normal (0, 0, 1) x (1, 0, 0)
  line L0 (0, 0) -> (0, 5.5) construction
  arc A0 (15.4415, 1.3095) -> (-15.4415, 1.3095) centre (0, 5.5) ccw
  line L1 (0, 0) -> (0, -5.5) construction
  arc A1 (-15.4415, -1.3095) -> (15.4415, -1.3095) centre (0, -5.5) ccw
  line L2 (0, 5.5) -> (0, -5.5) construction
  line L3 (-18.5, 5.5) -> (-18.5, -5.5)
  line L4 (18.5, -5.5) -> (18.5, 5.5)
  arc A2 (18.5, 5.5) -> (-18.5, 5.5) centre (0, 5.5) ccw
  arc A3 (-18.5, -5.5) -> (18.5, -5.5) centre (0, -5.5) ccw
  arc A4 (-15.4415, -1.3095) -> (-15.4415, 1.3095) centre (-20.267, 0) ccw
  arc A5 (15.4415, 1.3095) -> (15.4415, -1.3095) centre (20.267, 0) ccw
  dimension "d0" = 11
  dimension "d1" = 16
  dimension "d2" = 2.5
  dimension "d5" = 5
  dimension "d61" = 37
  constraints: 12 end point, 12 point on circle, 8 tangent, 6 centre point, 3 vertical, 2 coincident, 2 equal radius, 1 collinear, 1 midpoint, 1 parallel
  measures "d0" distance of L1.end L0.end
  measures "d1" radius of A0
  measures "d2" radial gap between concentric circles of A3 A1
  measures "d5" radius of A4
  measures "d61" distance between parallel lines of L4 L3
extrude "Extrusion1" add sketch "Sketch1" along normal mid plane 7
sketch "Sketch2" plane through (0, 0, -3.5) normal (0, 0, -1) x (-1, 0, 0)
  arc A0 (-18.5, -5.5) -> (18.5, -5.5) centre (0, -5.5) ccw
  line L0 (18.5, -5.5) -> (18.5, 5.5)
  arc A1 (18.5, 5.5) -> (-18.5, 5.5) centre (0, 5.5) ccw
  line L1 (-18.5, 5.5) -> (-18.5, -5.5)
  arc A2 (15.4415, 1.3095) -> (15.4415, -1.3095) centre (20.267, 0) ccw construction
  arc A3 (-15.4415, -1.3095) -> (15.4415, -1.3095) centre (0, -5.5) ccw construction
  arc A4 (-15.4415, -1.3095) -> (-15.4415, 1.3095) centre (-20.267, 0) ccw construction
  arc A5 (15.4415, 1.3095) -> (-15.4415, 1.3095) centre (0, 5.5) ccw construction
  point P0 (0, 0)
extrude "Extrusion2" add sketch "Sketch2" along normal blind 1.5
sketch "Sketch3" plane through (0, 0, -3.5) normal (0, 0, 1) x (1, 0, 0)
  circle A0 centre (0, 0) radius 3
  dimension "d8" = 6
  constraints: 1 centre point, 1 coincident
  measures "d8" diameter of A0
extrude "Extrusion3" cut sketch "Sketch3" against normal through all